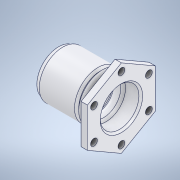
# Autodesk Inventor part: 22M_Standalone_Port_Hex_Lite_White
Saved by Autodesk Inventor 2020 (Build 240168000, 168)
## iProperties
Created: 2021-05-20
Part Number: 22M_Standalone_Port_Hex_Lite_White
Material: Generic
Document SubType Name: Modeling
Designer: Workshop
Density: 1 g/cm^3
Appearance: PTFE
Author: Workshop
Autodesk Inventor part; units mm, degrees
ref_plane "YZ Plane" through (0, 0, 0) normal (1, 0, 0) x (0, 1, 0)
ref_plane "XZ Plane" through (0, 0, 0) normal (0, 1, 0) x (-1, 0, 0)
ref_plane "XY Plane" through (0, 0, 0) normal (0, 0, 1) x (1, 0, 0)
sketch "Sketch1" plane through (0, 0, 0) normal (0, 0, 1) x (1, 0, 0)
  line L0 (0, 9.125) -> (0, 11.125)
  line L1 (0, 11.125) -> (18.6, 11.125)
  line L2 (18.6, 11.125) -> (19.6, 10.125)
  line L3 (19.6, 10.125) -> (20.6, 11.125)
  line L4 (20.6, 11.125) -> (26.6, 11.125)
  line L5 (0, 9.125) -> (16.781, 9.125)
  line L6 (16.781, 9.125) -> (19.6, 6.7596)
  line L7 (19.6, 6.7596) -> (22.419, 9.125)
  line L8 (22.419, 9.125) -> (29.5997, 9.125)
  line L9 (29.5997, 9.125) -> (29.5997, 20)
  line L10 (29.5997, 20) -> (26.6, 20)
  line L11 (26.6, 20) -> (26.6, 11.125)
  line L12 (-5.9199, 0) -> (35.5196, 0) projected
  point P0 (0, 0)
  dimension "d0" = 2
  dimension "d1" = 18.6
  dimension "d2" = 6
  dimension "d3" = 2
  dimension "d4" = 1
  dimension "d5" = 9.125
  dimension "d6" = 16.781
  dimension "d7" = 7.1807
  dimension "d8" = 50
  dimension "d9" = 20
  constraints: 24 end point, 4 perpendicular, 2 equal length, 2 horizontal, 2 point on line, 2 vertical alignment, 1 horizontal alignment, 1 vertical
  measures "d0" distance of L0.start L0.end
  measures "d1" distance of L0.end L1.end
  measures "d2" distance of L3.end L4.end
  measures "d3" distance of L3.end L1.end
  measures "d4" horizontal distance of L3.end L2.end
  measures "d5" distance of point (0, 0) L0.start
  measures "d6" distance of L0.start L5.end
  measures "d7" distance of L7.end L8.end
  measures "d8" angle of L9 L7
  measures "d9" distance from line of point (0, 0) L10
revolve "Revolution1" add sketch "Sketch1" angle 360 about axis through (-10, 0, 0) along (1, 0, 0)
fillet "Fillet1" radius 0.8 1 edges at (26.6, -11.125, 0)
sketch "Sketch2" plane through (29.5997, 0, 0) normal (1, 0, 0) x (0, 0, -1)
  circle A0 centre (0, -14.925) radius 1.6
  circle A1 centre (0, 0) radius 9.125 projected
  circle A2 centre (12.9254, -7.4625) radius 1.6
  circle A3 centre (12.9254, 7.4625) radius 1.6
  circle A4 centre (0, 14.925) radius 1.6
  circle A5 centre (-12.9254, 7.4625) radius 1.6
  circle A6 centre (-12.9254, -7.4625) radius 1.6
  line L0 (16, -9.2376) -> (0, -18.4752)
  line L1 (0, -18.4752) -> (-16, -9.2376)
  line L2 (-16, -9.2376) -> (-16, 9.2376)
  line L3 (-16, 9.2376) -> (0, 18.4752)
  line L4 (0, 18.4752) -> (16, 9.2376)
  line L5 (16, 9.2376) -> (16, -9.2376)
  circle A7 centre (0, 0) radius 20 projected
  point P0 (16, 0)
  dimension "d12" = 3.2
  dimension "d13" = 14.925
  dimension "d16" = 360
  dimension "d18" = 32
  constraints: 12 end point, 6 centre point, 1 coincident, 1 horizontal alignment, 1 midpoint, 1 vertical alignment, 26 other
  measures "d12" diameter of A0
  measures "d13" distance of point (0, 0) A0.centre
  measures "d18" distance between parallel lines of L2 L5
extrude "Extrusion1" cut sketch "Sketch2" against normal through all contours A0 | A2 | A3 | A4 | A5 | A6 | A7
fillet "Fillet2" radius 2.5 1 edges at (19.6, -6.7596, 0)
chamfer "Chamfer1" distance 2 distance2 0.875 1 edges at (0, -11.125, 0) measured on face at (0.5, -11.125, 0)
chamfer "Chamfer2" distance 0.875 angle 45 1 edges at (29.5997, -9.125, 0)
body "Solid1"
